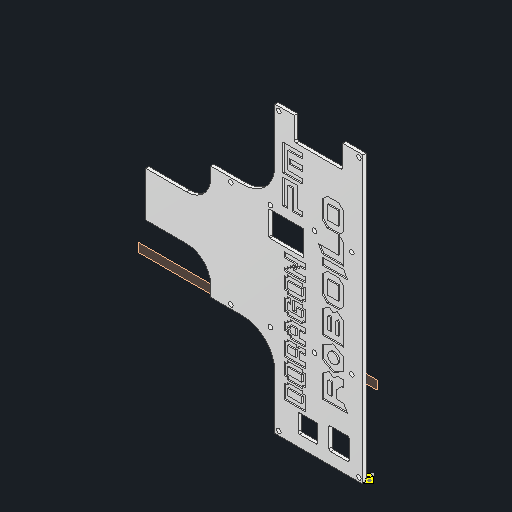
# Autodesk Inventor part: ceil
Saved by Autodesk Inventor 2023 (Build 270158000, 158)
## iProperties
Created: 2024-05-26
Part Number: ceil
Material: ABS Plastic
Document SubType Name: Modeling
Designer: szymo
Density: 1.06 g/cm^3
Appearance: Smooth - White
Mass: 25.7639 g
Surface Area: 285.339 cm^2
Volume: 24.3055 cm^3
TOTAL MASS: 0.0
Author: szymo
Autodesk Inventor part; units mm, degrees
ref_plane "YZ Plane" through (0, 0, 0) normal (1, 0, 0) x (0, 1, 0)
ref_plane "XZ Plane" through (0, 0, 0) normal (0, 1, 0) x (-1, 0, 0)
ref_plane "XY Plane" through (0, 0, 0) normal (0, 0, 1) x (1, 0, 0)
ref_plane "Work Plane1" through (-50.5, 0, 0) normal (0, 0, 1) x (1, 0, 0)
sketch "Sketch3" plane through (-50.5, 0, 0) normal (0, 0, 1) x (1, 0, 0)
  line L0 (0, 0) -> (135.5648, 0) projected
  line L1 (135.5648, 0) -> (135.5648, 5) projected
  line L2 (0, 5) -> (135.5648, 5) projected
  line L3 (0, 0) -> (0, 5) projected
  line L4 (0, 71) -> (135.5648, 71) projected
  line L5 (0, 71) -> (0, 66) projected
  line L6 (0, 66) -> (135.5648, 66) projected
  line L7 (135.5648, 71) -> (135.5648, 66) projected
  line L8 (131.5648, 119.5) -> (134.5648, 119.5) projected
  line L9 (135.5648, 124.5) -> (135.5648, 120.5) projected
  line L10 (135.5648, 124.5) -> (51.5, 124.5) projected
  line L11 (51.5, 123.5) -> (79.5, 123.5) projected
  line L12 (80.5, 122.5) -> (80.5, 120.5) projected
  line L13 (81.5, 119.5) -> (84.5, 119.5) projected
  line L14 (85.5, 122.5) -> (85.5, 120.5) projected
  line L15 (86.5, 123.5) -> (129.5648, 123.5) projected
  line L16 (130.5648, 122.5) -> (130.5648, 120.5) projected
  line L17 (120.8148, 112) -> (120.8148, 123) projected
  line L18 (120.8148, 123) -> (94.8148, 123) projected
  line L19 (94.8148, 123) -> (94.8148, 112) projected
  line L20 (94.8148, 112) -> (120.8148, 112) projected
  line L21 (130.5648, -51.5) -> (130.5648, -49.5) projected
  line L22 (51.5, -52.5) -> (79.5, -52.5) projected
  line L23 (85.5, -51.5) -> (85.5, -49.5) projected
  line L24 (131.5648, -48.5) -> (134.5648, -48.5) projected
  line L25 (80.5, -51.5) -> (80.5, -49.5) projected
  line L26 (86.5, -52.5) -> (129.5648, -52.5) projected
  line L27 (135.5648, -53.5) -> (51.5, -53.5) projected
  line L28 (135.5648, -53.5) -> (135.5648, -49.5) projected
  line L29 (81.5, -48.5) -> (84.5, -48.5) projected
  line L30 (95.5648, -45.8) -> (95.5648, -35.2) projected
  line L31 (106.8648, -35.2) -> (95.5648, -35.2) projected
  line L32 (106.8648, -35.2) -> (106.8648, -45.8) projected
  line L33 (95.5648, -45.8) -> (106.8648, -45.8) projected
  circle A0 centre (90.4898, -49.075) radius 1.675 projected
  circle A1 centre (124.5398, -49.075) radius 1.675 projected
  line L34 (126.3648, -33.5) -> (126.3648, -45.5) projected
  line L35 (126.3648, -45.5) -> (114.7648, -45.5) projected
  line L36 (114.7648, -45.5) -> (114.7648, -33.5) projected
  line L37 (114.7648, -33.5) -> (86.8648, -33.5) projected
  line L38 (86.8648, -33.5) -> (86.8648, -52.5) projected
  line L39 (86.8648, -52.5) -> (128.0648, -52.5) projected
  line L40 (128.0648, -52.5) -> (128.0648, -33.5) projected
  line L41 (128.0648, -33.5) -> (126.3648, -33.5) projected
  line L42 (126.3648, -32.7) -> (114.7648, -32.7) projected
  line L43 (114.7648, -32.7) -> (114.7648, -45.5) projected
  line L44 (114.7648, -45.5) -> (126.3648, -45.5) projected
  line L45 (126.3648, -45.5) -> (126.3648, -32.7) projected
  line L46 (80.5, -53.5) -> (135.5648, -53.5)
  line L47 (135.5648, -53.5) -> (135.5648, 124.5)
  line L48 (135.5648, 124.5) -> (80.5, 124.5)
  line L49 (80.5, 124.5) -> (80.5, -53.5)
  line L50 (0, 21.5) -> (80.5, 21.5)
  line L51 (80.5, 21.5) -> (80.5, 49.5)
  line L52 (80.5, 49.5) -> (0, 49.5)
  line L53 (0, 49.5) -> (0, 21.5)
  line L54 (80.5, 21.5) -> (50.5, 21.5)
  line L55 (50.5, 21.5) -> (50.5, 0)
  line L56 (50.5, 0) -> (80.5, 0)
  line L57 (80.5, 0) -> (80.5, 21.5)
  line L58 (80.5, 46.5815) -> (80.5, 71)
  line L59 (80.5, 71) -> (50.5, 71)
  line L60 (50.5, 71) -> (50.5, 49.5)
  arc A2 (97.9124, 50.9) -> (98.0124, 51) centre (97.9124, 51) ccw projected
  line L61 (77.4124, 50.9) -> (97.9124, 50.9) projected
  arc A3 (77.3124, 51) -> (77.4124, 50.9) centre (77.4124, 51) ccw projected
  line L62 (77.3124, 65.5) -> (77.3124, 51) projected
  arc A4 (77.4124, 65.6) -> (77.3124, 65.5) centre (77.4124, 65.5) ccw projected
  line L63 (97.9124, 65.6) -> (77.4124, 65.6) projected
  arc A5 (98.0124, 65.5) -> (97.9124, 65.6) centre (97.9124, 65.5) ccw projected
  line L64 (98.0124, 51) -> (98.0124, 65.5) projected
  line L65 (96.2124, 63.7) -> (96.2124, 52.8) projected
  arc A6 (96.2124, 63.7) -> (95.9124, 64) centre (95.9124, 63.7) ccw projected
  line L66 (95.9124, 64) -> (95.8124, 64) projected
  line L67 (95.8124, 64) -> (95.3509, 64.55) projected
  line L68 (95.3509, 64.55) -> (94.9739, 64.55) projected
  line L69 (94.9739, 64.55) -> (94.5124, 64) projected
  line L70 (94.5124, 64) -> (90.8124, 64) projected
  line L71 (90.8124, 64) -> (90.8124, 64.35) projected
  line L72 (90.8124, 64.35) -> (89.5124, 64.35) projected
  line L73 (89.5124, 64) -> (89.5124, 64.35) projected
  line L74 (89.5124, 64) -> (85.8124, 64) projected
  line L75 (85.8124, 64) -> (85.8124, 64.35) projected
  line L76 (85.8124, 64.35) -> (84.5124, 64.35) projected
  line L77 (84.5124, 64) -> (84.5124, 64.35) projected
  line L78 (84.5124, 64) -> (80.8124, 64) projected
  line L79 (80.8124, 64) -> (80.3509, 64.55) projected
  line L80 (80.3509, 64.55) -> (79.9739, 64.55) projected
  line L81 (79.9739, 64.55) -> (79.5124, 64) projected
  line L82 (79.5124, 64) -> (79.4124, 64) projected
  arc A7 (79.4124, 64) -> (79.1124, 63.7) centre (79.4124, 63.7) ccw projected
  line L83 (79.1124, 63.7) -> (79.1124, 52.8) projected
  arc A8 (79.1124, 52.8) -> (79.4124, 52.5) centre (79.4124, 52.8) ccw projected
  line L84 (79.4124, 52.5) -> (79.5124, 52.5) projected
  line L85 (79.5124, 52.5) -> (79.9739, 51.95) projected
  line L86 (80.3509, 51.95) -> (79.9739, 51.95) projected
  line L87 (80.3509, 51.95) -> (80.8124, 52.5) projected
  line L88 (80.8124, 52.5) -> (84.5124, 52.5) projected
  line L89 (84.5124, 52.5) -> (84.5124, 52.15) projected
  line L90 (85.8124, 52.15) -> (84.5124, 52.15) projected
  line L91 (85.8124, 52.5) -> (85.8124, 52.15) projected
  line L92 (85.8124, 52.5) -> (89.5124, 52.5) projected
  line L93 (89.5124, 52.5) -> (89.5124, 52.15) projected
  line L94 (90.8124, 52.15) -> (89.5124, 52.15) projected
  line L95 (90.8124, 52.5) -> (90.8124, 52.15) projected
  line L96 (90.8124, 52.5) -> (94.5124, 52.5) projected
  line L97 (94.5124, 52.5) -> (94.9739, 51.95) projected
  line L98 (95.3509, 51.95) -> (94.9739, 51.95) projected
  line L99 (95.3509, 51.95) -> (95.8124, 52.5) projected
  line L100 (95.8124, 52.5) -> (95.9124, 52.5) projected
  arc A9 (95.9124, 52.5) -> (96.2124, 52.8) centre (95.9124, 52.8) ccw projected
  line L101 (78.1624, 55.35) -> (78.8624, 55.35) projected
  line L102 (78.8624, 55.35) -> (78.8624, 61.15) projected
  line L103 (78.1624, 61.15) -> (78.8624, 61.15) projected
  line L104 (78.1624, 61.15) -> (78.1624, 55.35) projected
  line L105 (97.1624, 61.15) -> (97.1624, 55.35) projected
  line L106 (96.4624, 61.15) -> (97.1624, 61.15) projected
  line L107 (96.4624, 55.35) -> (96.4624, 61.15) projected
  line L108 (96.4624, 55.35) -> (97.1624, 55.35) projected
  arc A10 (76.8124, 51) -> (77.4124, 50.4) centre (77.4124, 51) ccw
  line L109 (77.4124, 50.4) -> (97.9124, 50.4)
  arc A11 (97.9124, 50.4) -> (98.5124, 51) centre (97.9124, 51) ccw
  line L110 (98.5124, 51) -> (98.5124, 65.5)
  arc A12 (98.5124, 65.5) -> (97.9124, 66.1) centre (97.9124, 65.5) ccw
  line L111 (97.9124, 66.1) -> (77.4124, 66.1)
  arc A13 (77.4124, 66.1) -> (76.8124, 65.5) centre (77.4124, 65.5) ccw
  line L112 (76.8124, 65.5) -> (76.8124, 51)
  line L113 (95.0648, -34.7) -> (95.0648, -46.3)
  line L114 (95.0648, -46.3) -> (107.3648, -46.3)
  line L115 (107.3648, -46.3) -> (107.3648, -34.7)
  line L116 (107.3648, -34.7) -> (95.0648, -34.7)
  line L117 (114.2648, -45.5) -> (114.2648, -32.2)
  line L118 (114.2648, -32.2) -> (126.8648, -32.2)
  line L119 (126.8648, -32.2) -> (126.8648, -45.5)
  line L120 (126.3648, -46) -> (114.7648, -46)
  line L121 (92.8148, 110) -> (92.8148, 125)
  line L122 (92.8148, 125) -> (122.8148, 125)
  line L123 (122.8148, 125) -> (122.8148, 110)
  line L124 (122.8148, 110) -> (92.8148, 110)
  line L125 (114.2648, -45.5) -> (114.2648, -46)
  line L126 (114.2648, -46) -> (114.7648, -46)
  line L127 (126.3648, -46) -> (126.8648, -46)
  line L128 (126.8648, -46) -> (126.8648, -45.5)
  line L129 (51.5, -53.5) -> (51.5, -52.5) projected
  line L130 (51.5, 124.5) -> (51.5, 123.5) projected
  circle A14 centre (105.3205, 68.5) radius 1.75 projected
  circle A15 centre (53, 68.5) radius 1.75 projected
  circle A16 centre (77.648, 2.5) radius 1.75 projected
  circle A17 centre (105.3205, 2.5) radius 1.75 projected
  circle A18 centre (53, 2.5) radius 1.75 projected
  circle A19 centre (128.5648, 2.5) radius 1.75 projected
  circle A20 centre (83, 122) radius 1.75 projected
  circle A21 centre (133.0648, 122) radius 1.75 projected
  arc A22 (130.5648, 120.5) -> (131.5648, 119.5) centre (131.5648, 120.5) ccw projected
  arc A23 (134.5648, 119.5) -> (135.5648, 120.5) centre (134.5648, 120.5) ccw projected
  arc A24 (80.5, 122.5) -> (79.5, 123.5) centre (79.5, 122.5) ccw projected
  arc A25 (86.5, 123.5) -> (85.5, 122.5) centre (86.5, 122.5) ccw projected
  arc A26 (130.5648, 122.5) -> (129.5648, 123.5) centre (129.5648, 122.5) ccw projected
  arc A27 (80.5, 120.5) -> (81.5, 119.5) centre (81.5, 120.5) ccw projected
  arc A28 (84.5, 119.5) -> (85.5, 120.5) centre (84.5, 120.5) ccw projected
  circle A29 centre (83, -51) radius 1.75 projected
  circle A30 centre (133.0648, -51) radius 1.75 projected
  arc A31 (131.5648, -48.5) -> (130.5648, -49.5) centre (131.5648, -49.5) ccw projected
  arc A32 (129.5648, -52.5) -> (130.5648, -51.5) centre (129.5648, -51.5) ccw projected
  arc A33 (85.5, -51.5) -> (86.5, -52.5) centre (86.5, -51.5) ccw projected
  arc A34 (79.5, -52.5) -> (80.5, -51.5) centre (79.5, -51.5) ccw projected
  arc A35 (135.5648, -49.5) -> (134.5648, -48.5) centre (134.5648, -49.5) ccw projected
  arc A36 (85.5, -49.5) -> (84.5, -48.5) centre (84.5, -49.5) ccw projected
  arc A37 (81.5, -48.5) -> (80.5, -49.5) centre (81.5, -49.5) ccw projected
  line L131 (50.5, 26.5) -> (0, 26.5) projected
  line L132 (0, 26.5) -> (0, 21.5) projected
  line L133 (50.5, 21.5) -> (0, 21.5) projected
  line L134 (50.5, 26.5) -> (50.5, 21.5) projected
  line L135 (50.5, 44.5) -> (0, 44.5) projected
  line L136 (50.5, 44.5) -> (50.5, 49.5) projected
  line L137 (50.5, 49.5) -> (0, 49.5) projected
  line L138 (0, 44.5) -> (0, 49.5) projected
  line L139 (50.5, 0) -> (40.5, 0)
  line L140 (40.5, 0) -> (40.5, 21.5)
  line L141 (40.5, 21.5) -> (50.5, 21.5)
  line L142 (50.5, 21.5) -> (50.5, 0)
  line L143 (50.5, 49.5) -> (40.5, 49.5)
  line L144 (40.5, 49.5) -> (40.5, 71)
  line L145 (40.5, 71) -> (50.5, 71)
  line L146 (50.5, 71) -> (50.5, 49.5)
  point P0 (80.5, -49.5)
  point P1 (80.5, -52.5)
  point P2 (122.8148, 124.5)
  point P3 (92.8148, 124.5)
  point P4 (80.5, 0)
  point P5 (0, 44)
  point P6 (50.5, 44)
  point P7 (122.8148, 124.5)
  point P8 (122.8148, 123.5)
  point P9 (92.8148, 123.5)
  point P10 (92.8148, 124.5)
  point P11 (80.5, 123.5)
  point P12 (50.5, 66)
  point P13 (50.5, 5)
  point P14 (80.5, -52.5)
  point P15 (80.5, 66)
  point P16 (80.5, 5)
  point P17 (50.5, 27)
  point P18 (0, 27)
  point P19 (135.5648, -49.5)
  point P20 (80.5, -49.5)
  point P21 (77.0807, 66)
  point P22 (80.5, 66.1)
  dimension "d16" = 0.5
  dimension "d17" = 0.5
  dimension "d18" = 0.5
  dimension "d19" = 0.5
  dimension "d20" = 2
  dimension "d191" = 10
  dimension "d192" = 10
  constraints: 84 end point, 11 parallel, 8 point on circle, 7 perpendicular, 6 horizontal, 5 point on line, 4 centre point, 4 vertical, 1 collinear, 21 other
  measures "d16" distance between parallel lines of L62 L112
  measures "d17" distance between parallel lines of L30 L113
  measures "d18" distance between parallel lines of L43 L117
  measures "d19" distance between parallel lines of L35 L120
  measures "d20" distance between parallel lines of L19 L121
  measures "d191" distance between parallel lines of L140 L55
  measures "d192" distance between parallel lines of L60 L144
extrude "Extrusion2" add sketch "Sketch3" along normal blind 2 contours L140 L2 L55 L0 | L55 L2 L49 L0 | L140 L50 L55 L2 | L49 L2 L1 L0 | L0 L47 A35 L24 A31 L21 A32 L26 L40 L41 L119 L118 L117 L37 L38 A33 L23 A36 L29 A37 L49 | L55 L50 L49 L2 | L50 L53 L131 L134 | A37 L29 A36 L23 A33 L26 A32 L21 A31 L24 A35 L28 L27 L49 L25 | L49 L109 A11 L110 A12 L6 L47 L2 | L134 L131 L53 L135 L136 L52 L49 L50 | L6 A12 L111 L49 L4 L7 | L53 L52 L136 L135 | L4 L49 A27 L13 A28 L14 A25 L15 L121 L124 L123 A26 L16 A22 L8 A23 L47 | L52 L60 L6 A13 L112 A10 L109 L49 | L49 L111 A13 L6 L60 L4 | A23 L8 A22 L16 A26 L15 L123 L10 L9 | L52 L144 L6 L60 | L60 L6 L144 L4 | L12 L49 L10 L121 L15 A25 L14 A28 L13 A27 | L38 L37 L117 L125 L126 L120 L127 L128 L119 L41 L40 L26 | A0 | A1 | A14 | A15 | A16 | A17 | A18 | A19 | A20 | A21 | A29 | A30
fillet "Fillet2" radius 1 10 edges at (44.5648, -46.3, 1) (44.5648, -34.7, 1) (56.8648, -34.7, 1) (56.8648, -46.3, 1) (63.7648, -46, 1) (63.7648, -32.2, 1) (76.3648, -32.2, 1) (76.3648, -46, 1) (42.3148, 110, 1) (72.3148, 110, 1)
fillet "Fillet3" radius 20 2 edges at (30, 0, 1) (30, 71, 1)
sketch "Sketch4" plane through (-50.5, 0, 2) normal (0, 0, 1) x (1, 0, 0)
  line L0 (130.5648, -51.5) -> (130.5648, -49.5) projected
  line L1 (51.5, -52.5) -> (79.5, -52.5) projected
  line L2 (85.5, -51.5) -> (85.5, -49.5) projected
  line L3 (131.5648, -48.5) -> (134.5648, -48.5) projected
  line L4 (80.5, -51.5) -> (80.5, -49.5) projected
  line L5 (86.5, -52.5) -> (129.5648, -52.5) projected
  line L6 (135.5648, -53.5) -> (51.5, -53.5) projected
  line L7 (135.5648, -53.5) -> (135.5648, -49.5) projected
  line L8 (81.5, -48.5) -> (84.5, -48.5) projected
  line L9 (131.5648, 119.5) -> (134.5648, 119.5) projected
  line L10 (135.5648, 124.5) -> (135.5648, 120.5) projected
  line L11 (135.5648, 124.5) -> (51.5, 124.5) projected
  line L12 (51.5, 123.5) -> (79.5, 123.5) projected
  line L13 (80.5, 122.5) -> (80.5, 120.5) projected
  line L14 (81.5, 119.5) -> (84.5, 119.5) projected
  line L15 (85.5, 122.5) -> (85.5, 120.5) projected
  line L16 (86.5, 123.5) -> (129.5648, 123.5) projected
  line L17 (130.5648, 122.5) -> (130.5648, 120.5) projected
  line L18 (51.5, 124.5) -> (51.5, 123.5) projected
  line L19 (51.5, -53.5) -> (51.5, -52.5) projected
  circle A0 centre (83, -51) radius 1.75 projected
  circle A1 centre (133.0648, -51) radius 1.75 projected
  arc A2 (131.5648, -48.5) -> (130.5648, -49.5) centre (131.5648, -49.5) ccw projected
  arc A3 (129.5648, -52.5) -> (130.5648, -51.5) centre (129.5648, -51.5) ccw projected
  arc A4 (85.5, -51.5) -> (86.5, -52.5) centre (86.5, -51.5) ccw projected
  arc A5 (79.5, -52.5) -> (80.5, -51.5) centre (79.5, -51.5) ccw projected
  arc A6 (135.5648, -49.5) -> (134.5648, -48.5) centre (134.5648, -49.5) ccw projected
  arc A7 (85.5, -49.5) -> (84.5, -48.5) centre (84.5, -49.5) ccw projected
  arc A8 (81.5, -48.5) -> (80.5, -49.5) centre (81.5, -49.5) ccw projected
  circle A9 centre (83, 122) radius 1.75 projected
  circle A10 centre (133.0648, 122) radius 1.75 projected
  arc A11 (130.5648, 120.5) -> (131.5648, 119.5) centre (131.5648, 120.5) ccw projected
  arc A12 (134.5648, 119.5) -> (135.5648, 120.5) centre (134.5648, 120.5) ccw projected
  arc A13 (80.5, 122.5) -> (79.5, 123.5) centre (79.5, 122.5) ccw projected
  arc A14 (86.5, 123.5) -> (85.5, 122.5) centre (86.5, 122.5) ccw projected
  arc A15 (130.5648, 122.5) -> (129.5648, 123.5) centre (129.5648, 122.5) ccw projected
  arc A16 (80.5, 120.5) -> (81.5, 119.5) centre (81.5, 120.5) ccw projected
  arc A17 (84.5, 119.5) -> (85.5, 120.5) centre (84.5, 120.5) ccw projected
  line L20 (50.5, 26.5) -> (0, 26.5) projected
  line L21 (0, 26.5) -> (0, 21.5) projected
  line L22 (50.5, 21.5) -> (0, 21.5) projected
  line L23 (50.5, 26.5) -> (50.5, 21.5) projected
  line L24 (50.5, 44.5) -> (0, 44.5) projected
  line L25 (50.5, 44.5) -> (50.5, 49.5) projected
  line L26 (50.5, 49.5) -> (0, 49.5) projected
  line L27 (0, 44.5) -> (0, 49.5) projected
  circle A18 centre (77.648, 68.5) radius 1.75 projected
  circle A19 centre (105.3205, 68.5) radius 1.75 projected
  circle A20 centre (53, 68.5) radius 1.75 projected
  circle A21 centre (128.5648, 68.5) radius 1.75 projected
  line L28 (0, 71) -> (135.5648, 71) projected
  line L29 (0, 71) -> (0, 66) projected
  line L30 (0, 66) -> (135.5648, 66) projected
  line L31 (135.5648, 71) -> (135.5648, 66) projected
  circle A22 centre (77.648, 2.5) radius 1.75 projected
  circle A23 centre (105.3205, 2.5) radius 1.75 projected
  circle A24 centre (53, 2.5) radius 1.75 projected
  circle A25 centre (128.5648, 2.5) radius 1.75 projected
  line L32 (0, 0) -> (135.5648, 0) projected
  line L33 (135.5648, 0) -> (135.5648, 5) projected
  line L34 (0, 5) -> (135.5648, 5) projected
  line L35 (0, 0) -> (0, 5) projected
  point P0 (50.5, 0)
  point P1 (0, 44)
  point P2 (50.5, 44)
  point P3 (50.5, 27)
  point P4 (0, 27)
  constraints: 12 coincident
hole "Hole2" at (32.5, -51, 2) at (82.5648, -51, 2) at (82.5648, 122, 2) at (32.5, 122, 2) at (54.8205, 68.5, 2) at (2.5, 2.5, 2) at (2.5, 68.5, 2) at (54.8205, 2.5, 2) at (78.0648, 2.5, 2) at (78.0648, 68.5, 2) at (27.148, 68.5, 2) at (27.148, 2.5, 2) direction (0, 0, -1) diameter 2.9 end through all clearance for "Countersunk Flat Head Screw ISO 2009/7046" size "M2.5" standard "ISO"
fillet "Fillet4" radius 15 2 edges at (-10, 21.5, 1) (-10, 49.5, 1)
sketch "Sketch5" plane through (-50.5, 0, 2) normal (0, 0, 1) x (1, 0, 0)
  line L0 (40.5, 0) -> (60.5, 0) projected
  line L1 (80.5, -53.5) -> (135.5648, -53.5) projected
  line L2 (135.5648, -53.5) -> (135.5648, 124.5) projected
  line L3 (135.5648, 124.5) -> (122.8148, 124.5) projected
  line L4 (122.8148, 124.5) -> (122.8148, 111) projected
  arc A0 (121.8148, 110) -> (122.8148, 111) centre (121.8148, 111) ccw projected
  line L5 (121.8148, 110) -> (93.8148, 110) projected
  arc A1 (92.8148, 111) -> (93.8148, 110) centre (93.8148, 111) ccw projected
  line L6 (92.8148, 111) -> (92.8148, 124.5) projected
  line L7 (92.8148, 124.5) -> (80.5, 124.5) projected
  line L8 (60.5, 71) -> (40.5, 71) projected
  line L9 (25.5, 49.5) -> (0, 49.5) projected
  line L10 (0, 49.5) -> (0, 21.5) projected
  line L11 (0, 21.5) -> (25.5, 21.5) projected
  line L12 (77.4124, 66.1) -> (97.9124, 66.1) projected
  arc A2 (98.5124, 65.5) -> (97.9124, 66.1) centre (97.9124, 65.5) ccw projected
  line L13 (98.5124, 65.5) -> (98.5124, 51) projected
  arc A3 (97.9124, 50.4) -> (98.5124, 51) centre (97.9124, 51) ccw projected
  line L14 (97.9124, 50.4) -> (77.4124, 50.4) projected
  arc A4 (76.8124, 51) -> (77.4124, 50.4) centre (77.4124, 51) ccw projected
  line L15 (76.8124, 51) -> (76.8124, 65.5) projected
  arc A5 (77.4124, 66.1) -> (76.8124, 65.5) centre (77.4124, 65.5) ccw projected
  line L16 (114.2648, -45) -> (114.2648, -33.2) projected
  arc A6 (115.2648, -32.2) -> (114.2648, -33.2) centre (115.2648, -33.2) ccw projected
  line L17 (115.2648, -32.2) -> (125.8648, -32.2) projected
  arc A7 (126.8648, -33.2) -> (125.8648, -32.2) centre (125.8648, -33.2) ccw projected
  line L18 (126.8648, -33.2) -> (126.8648, -45) projected
  arc A8 (125.8648, -46) -> (126.8648, -45) centre (125.8648, -45) ccw projected
  line L19 (125.8648, -46) -> (115.2648, -46) projected
  arc A9 (114.2648, -45) -> (115.2648, -46) centre (115.2648, -45) ccw projected
  line L20 (96.0648, -34.7) -> (106.3648, -34.7) projected
  arc A10 (107.3648, -35.7) -> (106.3648, -34.7) centre (106.3648, -35.7) ccw projected
  line L21 (107.3648, -35.7) -> (107.3648, -45.3) projected
  arc A11 (106.3648, -46.3) -> (107.3648, -45.3) centre (106.3648, -45.3) ccw projected
  line L22 (106.3648, -46.3) -> (96.0648, -46.3) projected
  arc A12 (95.0648, -45.3) -> (96.0648, -46.3) centre (96.0648, -45.3) ccw projected
  line L23 (95.0648, -45.3) -> (95.0648, -35.7) projected
  arc A13 (96.0648, -34.7) -> (95.0648, -35.7) centre (96.0648, -35.7) ccw projected
  line L24 (105.3205, -31.7) -> (105.3205, 48.4) construction
  line L25 (105.3205, 48.4) -> (80.5, 48.4) construction
  line L26 (80.5, 48.4) -> (80.5, -31.7) construction
  line L27 (80.5, -31.7) -> (105.3205, -31.7) construction
  line L28 (110.1651, 28.6458) -> (110.1651, 14.5717) projected
  line L29 (119.2148, -10.52) -> (122.2141, -7.4431) projected
  line L30 (122.2141, -7.4431) -> (123.5648, -7.4431) projected
  line L31 (123.5648, -7.4431) -> (123.5648, -3.1151) projected
  line L32 (123.5648, -3.1151) -> (119.5551, -3.1151) projected
  line L33 (119.5551, -3.1151) -> (117.3584, -5.3021) projected
  line L34 (117.3584, -5.3021) -> (114.3535, -3.0659) projected
  line L35 (114.3535, -3.0659) -> (110.1651, -6.1782) projected
  line L36 (110.1651, -6.1782) -> (110.1651, -20.0711) projected
  line L37 (110.1651, -20.0711) -> (125.9602, -20.0711) projected
  line L38 (125.9602, -20.0711) -> (123.4807, -15.7431) projected
  line L39 (123.4807, -15.7431) -> (119.2148, -15.7431) projected
  line L40 (119.2148, -15.7431) -> (119.2148, -10.52) projected
  line L41 (114.6271, -7.6036) -> (115.8612, -8.5098) projected
  line L42 (115.8612, -8.5098) -> (115.8612, -15.7431) projected
  line L43 (115.8612, -15.7431) -> (113.4584, -15.7431) projected
  line L44 (113.4584, -15.7431) -> (113.4584, -8.4973) projected
  line L45 (113.4584, -8.4973) -> (114.6271, -7.6036) projected
  line L46 (123.5648, 1.4254) -> (123.5648, 9.1617) projected
  line L47 (123.5648, 9.1617) -> (116.8649, 13.0299) projected
  line L48 (116.8649, 13.0299) -> (110.1651, 9.1617) projected
  line L49 (110.1651, 9.1617) -> (110.1651, 1.4254) projected
  line L50 (110.1651, 1.4254) -> (116.8649, -2.4427) projected
  line L51 (116.8649, -2.4427) -> (123.5648, 1.4254) projected
  circle A14 centre (116.8649, 5.2936) radius 3.3 projected
  line L52 (123.5848, 14.5717) -> (123.5848, 28.6458) projected
  line L53 (123.5848, 28.6458) -> (119.3867, 31.747) projected
  line L54 (119.3867, 31.747) -> (116.875, 29.8983) projected
  line L55 (116.875, 29.8983) -> (114.3632, 31.747) projected
  line L56 (114.3632, 31.747) -> (110.1651, 28.6458) projected
  line L57 (110.1651, 28.6458) -> (110.1651, 14.5717) projected
  line L58 (110.1651, 14.5717) -> (123.5848, 14.5717) projected
  line L59 (115.3489, 26.1486) -> (115.3489, 18.8997) projected
  line L60 (115.3489, 18.8997) -> (113.4785, 18.8997) projected
  line L61 (113.4785, 18.8997) -> (113.4785, 26.1539) projected
  line L62 (113.4785, 26.1539) -> (114.3691, 26.9374) projected
  line L63 (114.3691, 26.9374) -> (115.3489, 26.1486) projected
  line L64 (118.4011, 18.8997) -> (118.4011, 26.1486) projected
  line L65 (118.4011, 26.1486) -> (119.3808, 26.9374) projected
  line L66 (119.3808, 26.9374) -> (120.2715, 26.1539) projected
  line L67 (120.2715, 26.1539) -> (120.2715, 18.8997) projected
  line L68 (120.2715, 18.8997) -> (118.4011, 18.8997) projected
  line L69 (120.494, 33.3579) -> (123.5648, 36.4286) projected
  line L70 (123.5648, 36.4286) -> (123.5648, 47.4441) projected
  line L71 (123.5648, 47.4441) -> (120.494, 50.5148) projected
  line L72 (120.494, 50.5148) -> (113.2358, 50.5148) projected
  line L73 (113.2358, 50.5148) -> (110.1651, 47.4441) projected
  line L74 (110.1651, 47.4441) -> (110.1651, 36.4286) projected
  line L75 (110.1651, 36.4286) -> (113.2358, 33.3579) projected
  line L76 (113.2358, 33.3579) -> (120.494, 33.3579) projected
  line L77 (120.2715, 37.686) -> (113.4584, 37.686) projected
  line L78 (113.4584, 37.686) -> (113.4584, 46.1868) projected
  line L79 (113.4584, 46.1868) -> (120.2715, 46.1868) projected
  line L80 (120.2715, 46.1868) -> (120.2715, 37.686) projected
  line L81 (125.9586, 52.2145) -> (123.5013, 56.5425) projected
  line L82 (123.5013, 56.5425) -> (110.1651, 56.5425) projected
  line L83 (110.1651, 56.5425) -> (110.1651, 52.2145) projected
  line L84 (110.1651, 52.2145) -> (125.9586, 52.2145) projected
  line L85 (123.5648, 88.0003) -> (120.494, 91.071) projected
  line L86 (120.494, 91.071) -> (113.2358, 91.071) projected
  line L87 (113.2358, 91.071) -> (110.1651, 88.0003) projected
  line L88 (110.1651, 88.0003) -> (110.1651, 76.9848) projected
  line L89 (110.1651, 76.9848) -> (113.2358, 73.9141) projected
  line L90 (113.2358, 73.9141) -> (120.2715, 73.9141) projected
  line L91 (120.2715, 73.9141) -> (120.2715, 62.7008) projected
  line L92 (120.2715, 62.7008) -> (107.738, 62.7008) projected
  line L93 (107.738, 62.7008) -> (110.2396, 58.3727) projected
  line L94 (110.2396, 58.3727) -> (123.5848, 58.3727) projected
  line L95 (123.5848, 58.3727) -> (123.5848, 70.8415) projected
  line L96 (123.5848, 70.8415) -> (120.5032, 73.9232) projected
  line L97 (120.5032, 73.9232) -> (123.5648, 76.9848) projected
  line L98 (123.5648, 76.9848) -> (123.5648, 88.0003) projected
  line L99 (120.2715, 78.2421) -> (113.4584, 78.2421) projected
  line L100 (113.4584, 78.2421) -> (113.4584, 86.743) projected
  line L101 (113.4584, 86.743) -> (120.2715, 86.743) projected
  line L102 (120.2715, 86.743) -> (120.2715, 78.2421) projected
  line L103 (91.5024, 71.975) -> (97.5262, 71.975) projected
  line L104 (97.5262, 71.975) -> (97.5262, 74.9242) projected
  line L105 (97.5262, 74.9242) -> (94.45, 74.9242) projected
  line L106 (94.45, 74.9242) -> (94.45, 87.525) projected
  line L107 (94.45, 87.525) -> (85.5, 87.525) projected
  line L108 (85.5, 87.525) -> (85.5, 71.975) projected
  line L109 (85.5, 71.975) -> (88.675, 71.975) projected
  line L110 (88.675, 71.975) -> (88.675, 84.4887) projected
  line L111 (88.675, 84.4887) -> (91.5024, 84.4887) projected
  line L112 (91.5024, 84.4887) -> (91.5024, 71.975) projected
  line L113 (85.5, 106.5) -> (85.5, 89.825) projected
  line L114 (85.5, 89.825) -> (97.6, 89.825) projected
  line L115 (97.6, 89.825) -> (97.6, 92.775) projected
  line L116 (97.6, 92.775) -> (88.6, 92.775) projected
  line L117 (88.6, 92.775) -> (88.6, 103.4705) projected
  line L118 (88.6, 103.4705) -> (97.5254, 103.4705) projected
  line L119 (97.5254, 103.4705) -> (97.5254, 106.5) projected
  line L120 (97.5254, 106.5) -> (85.5, 106.5) projected
  line L121 (89.7, 99.675) -> (89.7, 96.575) projected
  line L122 (89.7, 96.575) -> (97.6, 96.575) projected
  line L123 (97.6, 96.575) -> (97.6, 99.675) projected
  line L124 (97.6, 99.675) -> (89.7, 99.675) projected
  line L125 (80.5, -20) -> (80.5, -53.5) projected
  line L126 (80.5, 124.5) -> (80.5, 91) projected
  arc A15 (80.5, -20) -> (60.5, 0) centre (60.5, -20) ccw projected
  arc A16 (60.5, 71) -> (80.5, 91) centre (60.5, 91) ccw projected
  circle A17 centre (105.3205, 2.5) radius 1.45 projected
  line L127 (40.5, 71) -> (40.5, 64.5) projected
  line L128 (40.5, 6.5) -> (40.5, 0) projected
  arc A18 (25.5, 49.5) -> (40.5, 64.5) centre (25.5, 64.5) ccw projected
  arc A19 (40.5, 6.5) -> (25.5, 21.5) centre (25.5, 6.5) ccw projected
  line L129 (99.4102, -32.275) -> (86.4102, -32.275)
  line L130 (86.4102, -32.275) -> (86.4102, -23.4821)
  line L131 (86.4102, -23.4821) -> (88.2317, -23.4821)
  line L132 (88.2317, -23.4821) -> (88.2317, -22.0607)
  line L133 (88.2317, -22.0607) -> (97.5888, -22.0607)
  line L134 (97.5888, -22.0607) -> (97.5888, -23.4821)
  line L135 (97.5888, -23.4821) -> (99.4102, -23.4821)
  line L136 (99.4102, -23.4821) -> (99.4102, -32.275)
  line L137 (97.3317, -25.1679) -> (88.4888, -25.1679)
  line L138 (88.4888, -25.1679) -> (88.4888, -29.1679)
  line L139 (88.4888, -29.1679) -> (97.3317, -29.1679)
  line L140 (97.3317, -29.1679) -> (97.3317, -25.1679)
  line L141 (99.4102, -19.2464) -> (97.5888, -19.2464)
  line L142 (97.5888, -19.2464) -> (97.5888, -20.6679)
  line L143 (97.5888, -20.6679) -> (88.2317, -20.6679)
  line L144 (88.2317, -20.6679) -> (88.2317, -19.2464)
  line L145 (88.2317, -19.2464) -> (86.4102, -19.2464)
  line L146 (86.4102, -19.2464) -> (86.4102, -11.875)
  line L147 (86.4102, -11.875) -> (88.2317, -11.875)
  line L148 (88.2317, -11.875) -> (88.2317, -10.4536)
  line L149 (88.2317, -10.4536) -> (97.5888, -10.4536)
  line L150 (97.5888, -10.4536) -> (97.5888, -11.875)
  line L151 (97.5888, -11.875) -> (99.4102, -11.875)
  line L152 (99.4102, -11.875) -> (99.4102, -19.2464)
  line L153 (97.3317, -13.5607) -> (88.4888, -13.5607)
  line L154 (88.4888, -13.5607) -> (88.4888, -17.5607)
  line L155 (88.4888, -17.5607) -> (97.3317, -17.5607)
  line L156 (97.3317, -17.5607) -> (97.3317, -13.5607)
  line L157 (99.4102, -9.0607) -> (86.4102, -9.0607)
  line L158 (86.4102, -9.0607) -> (86.4102, -0.2679)
  line L159 (86.4102, -0.2679) -> (88.2317, -0.2679)
  line L160 (88.2317, -0.2679) -> (88.2317, 1.1536)
  line L161 (88.2317, 1.1536) -> (93.9531, 1.1536)
  line L162 (93.9531, 1.1536) -> (93.9531, -0.2679)
  line L163 (93.9531, -0.2679) -> (95.5102, -0.2679)
  line L164 (95.5102, -0.2679) -> (95.5102, 1.1536)
  line L165 (95.5102, 1.1536) -> (99.4102, 1.1536)
  line L166 (99.4102, 1.1536) -> (99.4102, -1.9536)
  line L167 (99.4102, -1.9536) -> (95.7674, -1.9536)
  line L168 (95.7674, -1.9536) -> (95.7674, -5.9536)
  line L169 (95.7674, -5.9536) -> (99.4102, -5.9536)
  line L170 (99.4102, -5.9536) -> (99.4102, -9.0607)
  line L171 (93.6959, -1.9536) -> (88.4888, -1.9536)
  line L172 (88.4888, -1.9536) -> (88.4888, -5.9536)
  line L173 (88.4888, -5.9536) -> (93.6959, -5.9536)
  line L174 (93.6959, -5.9536) -> (93.6959, -1.9536)
  line L175 (99.4102, 2.5464) -> (90.0531, 2.5464)
  line L176 (90.0531, 2.5464) -> (90.0531, 3.9679)
  line L177 (90.0531, 3.9679) -> (88.2317, 3.9679)
  line L178 (88.2317, 3.9679) -> (88.2317, 5.3893)
  line L179 (88.2317, 5.3893) -> (86.4102, 5.3893)
  line L180 (86.4102, 5.3893) -> (86.4102, 9.9179)
  line L181 (86.4102, 9.9179) -> (88.2317, 9.9179)
  line L182 (88.2317, 9.9179) -> (88.2317, 11.3393)
  line L183 (88.2317, 11.3393) -> (90.0531, 11.3393)
  line L184 (90.0531, 11.3393) -> (90.0531, 12.7607)
  line L185 (90.0531, 12.7607) -> (99.4102, 12.7607)
  line L186 (99.4102, 12.7607) -> (99.4102, 9.6536)
  line L187 (99.4102, 9.6536) -> (95.7674, 9.6536)
  line L188 (95.7674, 9.6536) -> (95.7674, 5.6536)
  line L189 (95.7674, 5.6536) -> (99.4102, 5.6536)
  line L190 (99.4102, 5.6536) -> (99.4102, 2.5464)
  line L191 (93.6959, 9.6536) -> (90.3102, 9.6536)
  line L192 (90.3102, 9.6536) -> (90.3102, 8.2321)
  line L193 (90.3102, 8.2321) -> (88.4888, 8.2321)
  line L194 (88.4888, 8.2321) -> (88.4888, 7.075)
  line L195 (88.4888, 7.075) -> (90.3102, 7.075)
  line L196 (90.3102, 7.075) -> (90.3102, 5.6536)
  line L197 (90.3102, 5.6536) -> (93.6959, 5.6536)
  line L198 (93.6959, 5.6536) -> (93.6959, 9.6536)
  line L199 (99.4102, 15.575) -> (97.5888, 15.575)
  line L200 (97.5888, 15.575) -> (97.5888, 14.1536)
  line L201 (97.5888, 14.1536) -> (88.2317, 14.1536)
  line L202 (88.2317, 14.1536) -> (88.2317, 15.575)
  line L203 (88.2317, 15.575) -> (86.4102, 15.575)
  line L204 (86.4102, 15.575) -> (86.4102, 22.9464)
  line L205 (86.4102, 22.9464) -> (88.2317, 22.9464)
  line L206 (88.2317, 22.9464) -> (88.2317, 24.3679)
  line L207 (88.2317, 24.3679) -> (90.3102, 24.3679)
  line L208 (90.3102, 24.3679) -> (90.3102, 21.2607)
  line L209 (90.3102, 21.2607) -> (88.4888, 21.2607)
  line L210 (88.4888, 21.2607) -> (88.4888, 17.2607)
  line L211 (88.4888, 17.2607) -> (97.3317, 17.2607)
  line L212 (97.3317, 17.2607) -> (97.3317, 21.2607)
  line L213 (97.3317, 21.2607) -> (93.9531, 21.2607)
  line L214 (93.9531, 21.2607) -> (93.9531, 18.4179)
  line L215 (93.9531, 18.4179) -> (91.8745, 18.4179)
  line L216 (91.8745, 18.4179) -> (91.8745, 24.3679)
  line L217 (91.8745, 24.3679) -> (97.5888, 24.3679)
  line L218 (97.5888, 24.3679) -> (97.5888, 22.9464)
  line L219 (97.5888, 22.9464) -> (99.4102, 22.9464)
  line L220 (99.4102, 22.9464) -> (99.4102, 15.575)
  line L221 (99.4102, 27.1821) -> (97.5888, 27.1821)
  line L222 (97.5888, 27.1821) -> (97.5888, 25.7607)
  line L223 (97.5888, 25.7607) -> (88.2317, 25.7607)
  line L224 (88.2317, 25.7607) -> (88.2317, 27.1821)
  line L225 (88.2317, 27.1821) -> (86.4102, 27.1821)
  line L226 (86.4102, 27.1821) -> (86.4102, 34.5536)
  line L227 (86.4102, 34.5536) -> (88.2317, 34.5536)
  line L228 (88.2317, 34.5536) -> (88.2317, 35.975)
  line L229 (88.2317, 35.975) -> (97.5888, 35.975)
  line L230 (97.5888, 35.975) -> (97.5888, 34.5536)
  line L231 (97.5888, 34.5536) -> (99.4102, 34.5536)
  line L232 (99.4102, 34.5536) -> (99.4102, 27.1821)
  line L233 (97.3317, 32.8679) -> (88.4888, 32.8679)
  line L234 (88.4888, 32.8679) -> (88.4888, 28.8679)
  line L235 (88.4888, 28.8679) -> (97.3317, 28.8679)
  line L236 (97.3317, 28.8679) -> (97.3317, 32.8679)
  line L237 (99.4102, 44.475) -> (95.7674, 44.475)
  line L238 (95.7674, 44.475) -> (95.7674, 43.0536)
  line L239 (95.7674, 43.0536) -> (93.6959, 43.0536)
  line L240 (93.6959, 43.0536) -> (93.6959, 44.475)
  line L241 (93.6959, 44.475) -> (86.4102, 44.475)
  line L242 (86.4102, 44.475) -> (86.4102, 47.5821)
  line L243 (86.4102, 47.5821) -> (99.4102, 47.5821)
  line L244 (99.4102, 47.5821) -> (99.4102, 44.475)
  line L245 (99.4102, 37.3679) -> (86.4102, 37.3679)
  line L246 (86.4102, 37.3679) -> (86.4102, 39.0536)
  line L247 (86.4102, 39.0536) -> (88.2317, 39.0536)
  line L248 (88.2317, 39.0536) -> (88.2317, 40.475)
  line L249 (88.2317, 40.475) -> (90.0531, 40.475)
  line L250 (90.0531, 40.475) -> (90.0531, 41.8964)
  line L251 (90.0531, 41.8964) -> (92.1317, 41.8964)
  line L252 (92.1317, 41.8964) -> (92.1317, 40.475)
  line L253 (92.1317, 40.475) -> (99.4102, 40.475)
  line L254 (99.4102, 40.475) -> (99.4102, 37.3679)
  line L255 (93.9531, 41.6321) -> (91.8745, 41.6321)
  line L256 (91.8745, 41.6321) -> (91.8745, 43.3179)
  line L257 (91.8745, 43.3179) -> (93.9531, 43.3179)
  line L258 (93.9531, 43.3179) -> (93.9531, 41.6321)
  point P0 (50.5, 0)
  dimension "d188" = 3
  dimension "d189" = 2
  constraints: 2 point on line, 2 other
  measures "d188" distance between parallel lines of L20 L27
  measures "d189" distance between parallel lines of L14 L25
extrude "Extrusion4" cut sketch "Sketch5" against normal blind 0.8 contours L56 L55 L54 L53 L52 L58 L28 | L40 L39 L38 L37 L36 L35 L34 L33 L32 L31 L30 L29 | L51 L50 L49 L48 L47 L46 | L76 L75 L74 L73 L72 L71 L70 L69 | L84 L83 L82 L81 | L98 L97 L96 L95 L94 L93 L92 L91 L90 L89 L88 L87 L86 L85 | L112 L111 L110 L109 L108 L107 L106 L105 L104 L103 | L120 L119 L118 L117 L116 L115 L114 L113 | L124 L123 L122 L121 | L129 L130 L131 L132 L133 L134 L135 L136 | L141 L142 L143 L144 L145 L146 L147 L148 L149 L150 L151 L152 | L157 L158 L159 L160 L161 L162 L163 L164 L165 L166 L167 L168 L169 L170 | L175 L176 L177 L178 L179 L180 L181 L182 L183 L184 L185 L186 L187 L188 L189 L190 | L199 L200 L201 L202 L203 L204 L205 L206 L207 L208 L209 L210 L211 L212 L213 L214 L215 L216 L217 L218 L219 L220 | L221 L222 L223 L224 L225 L226 L227 L228 L229 L230 L231 L232 | L237 L238 L239 L258 L257 L240 L241 L242 L243 L244 | L258 L255 L252 L251 L256 L257 L240 L239 | L239 L240 L257 L258 | L255 L256 L251 L252 | L252 L253 L254 L245 L246 L247 L248 L249 L250 L251 L256 L255
body "Solid2"
